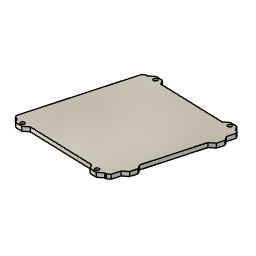
Arc Bed (Mandala) - BETA (Autodesk Fusion 360 design; units mm, degrees)
Autodesk Fusion 360 part; units mm, degrees
note: some values were not read from the file. Set by a fixed rule: which sketch regions a step uses.
sketch "Sketch1" plane through (0, 0, 0) normal (0, 0, 1) x (1, 0, 0) in component "Precision Alca5/ATP5/MIC6/5083 Aluminum Bed Plate"
  line L0 (92.5, -92.5) -> (-92.5, -92.5)
  line L1 (-92.5, -92.5) -> (-92.5, 92.5)
  line L2 (92.5, 92.5) -> (92.5, -92.5)
  line L3 (92.5, -92.5) -> (-92.5, 92.5) construction
  line L4 (-92.5, -92.5) -> (92.5, 92.5) construction
  line L5 (-88.5, 92.5) -> (-92.5, 88.5)
  line L6 (88.5, 92.5) -> (92.5, 88.5)
  line L7 (72.5, -72.5) -> (-72.5, -72.5) construction
  line L8 (-72.5, -72.5) -> (-72.5, 72.5) construction
  line L9 (-72.5, 72.5) -> (72.5, 72.5) construction
  line L10 (72.5, 72.5) -> (72.5, -72.5) construction
  line L11 (72.5, -72.5) -> (-72.5, 72.5) construction
  line L12 (-72.5, -72.5) -> (72.5, 72.5) construction
  circle A0 centre (72.5, 72.5) radius 9.575
  circle A1 centre (-72.5, 72.5) radius 9.575
  circle A2 centre (-72.5, -72.5) radius 9.575
  circle A3 centre (72.5, -72.5) radius 9.575
  line L13 (-92.5, -92.5) -> (-92.5, -99.5)
  line L14 (-92.5, -99.5) -> (92.5, -99.5)
  line L15 (92.5, -99.5) -> (92.5, -92.5)
  line L16 (-92.5, -74.5) -> (-67.5, -99.5)
  line L17 (92.5, -74.5) -> (67.5, -99.5)
  line L18 (-55.5, -99.5) -> (-48.5, -92.5)
  line L19 (55.5, -99.5) -> (48.5, -92.5)
  line L20 (-92.5, -88.5) -> (-88.5, -92.5)
  line L21 (92.5, -88.5) -> (88.5, -92.5)
  line L22 (90, 90) -> (-90, 90)
  line L23 (-90, 90) -> (-90, -90)
  line L24 (-90, -90) -> (90, -90)
  line L25 (90, -90) -> (90, 90)
  line L26 (90, 90) -> (-90, -90) construction
  line L27 (-90, 90) -> (90, -90) construction
  line L28 (-89.5, -89.5) -> (89.5, -89.5)
  line L29 (89.5, -89.5) -> (89.5, 89.5)
  line L30 (89.5, 89.5) -> (-89.5, 89.5)
  line L31 (-89.5, 89.5) -> (-89.5, -89.5)
  line L32 (-70, 90) -> (-70, 89.5)
  line L33 (-89.5, 70) -> (-90, 70)
  line L34 (-90, -70) -> (-89.5, -70)
  line L35 (-70, -89.5) -> (-70, -90)
  line L36 (70, -89.5) -> (70, -90)
  line L37 (89.5, -70) -> (90, -70)
  line L38 (70, 90) -> (70, 89.5)
  line L39 (89.5, 70) -> (90, 70)
  line L40 (-92.5, 72.5) -> (-99.5, 72.5) construction
  line L41 (-99.5, 78.5) -> (-99.5, 66.5)
  line L42 (-99.5, 78.5) -> (-92.5, 85.5)
  line L43 (-92.5, 72.5) -> (-72.5, 72.5) construction
  line L44 (-92.5, 59.5) -> (-99.5, 66.5)
  circle A4 centre (-94.05, 72.5) radius 1.55
  line L45 (-72.5, 0) -> (72.5, 0)
  line L46 (0, 72.5) -> (0, -72.5)
  circle A5 centre (-94.05, 72.5) radius 3.1
  circle A6 centre (-94.05, -72.5) radius 1.55
  circle A7 centre (-94.05, -72.5) radius 3.1
  line L47 (-92.5, -59.5) -> (-99.5, -66.5)
  line L48 (-99.5, -78.5) -> (-99.5, -66.5)
  line L49 (-99.5, -78.5) -> (-92.5, -85.5)
  circle A8 centre (94.05, -72.5) radius 1.55
  circle A9 centre (94.05, -72.5) radius 3.1
  line L50 (99.5, -78.5) -> (99.5, -66.5)
  line L51 (99.5, -78.5) -> (92.5, -85.5)
  line L52 (92.5, -59.5) -> (99.5, -66.5)
  circle A10 centre (94.05, 72.5) radius 1.55
  circle A11 centre (94.05, 72.5) radius 3.1
  line L53 (92.5, 59.5) -> (99.5, 66.5)
  line L54 (99.5, 78.5) -> (99.5, 66.5)
  line L55 (99.5, 78.5) -> (92.5, 85.5)
  circle A12 centre (-72.5, 0) radius 9.575
  circle A13 centre (0, 0) radius 9.575
  circle A14 centre (0, 72.5) radius 9.575
  circle A15 centre (72.5, 0) radius 9.575
  circle A16 centre (0, -72.5) radius 9.575
  line L56 (-1.6, 25.2701) -> (-1.6, 28.4701) construction
  line L57 (-1.6, 28.4701) -> (1.6, 28.4701) construction
  line L58 (1.6, 25.2701) -> (-1.6, 28.4701) construction
  line L59 (-1.6, 25.2701) -> (1.6, 28.4701) construction
  line L60 (92.5, 92.5) -> (-88.5, 92.5)
  line L61 (1.6, 28.4701) -> (1.6, 25.2701) construction
  line L62 (-1.6, 25.2701) -> (1.6, 25.2701) construction
  circle A17 centre (0, 26.8701) radius 2.2627
  line L63 (0, 26.8701) -> (-65.6299, 92.5) construction
  circle A18 centre (-11.3137, 38.1838) radius 2.2627
  line L64 (-1.6, 25.2701) -> (-12.9137, 36.5838)
  line L65 (1.6, 28.4701) -> (-9.7137, 39.7838)
  line L66 (-92.5, 92.5) -> (-88.5, 92.5)
  line L67 (-13.4561, 38.9119) -> (-67.0442, 92.5)
  line L68 (-12.0419, 40.3261) -> (-64.2157, 92.5)
  point P0 (0, 26.8701)
  dimension "d434_1" = 185
  dimension "d435_1" = 185
  dimension "d437_1" = 4
  dimension "d438_1" = 4
  dimension "d443_1" = 145
  dimension "d444_1" = 145
  dimension "d445_1" = 19.15
  dimension "d448_1" = 19.15
  dimension "d451_1" = 19.15
  dimension "d452_1" = 19.15
  dimension "d471_1" = 7
  dimension "d472_1" = 25
  dimension "d473_1" = 25
  dimension "d479_1" = 12
  dimension "d480_1" = 12
  dimension "d481_1" = 135
  dimension "d482_1" = 135
  dimension "d561_1" = 4
  dimension "d562_1" = 4
  dimension "d574_1" = 180
  dimension "d575_1" = 180
  dimension "d577_1" = 20
  dimension "d578_1" = 20
  dimension "d581_1" = 20
  dimension "d582_1" = 20
  dimension "d583_1" = 20
  dimension "d584_1" = 20
  dimension "d585_1" = 20
  dimension "d586_1" = 20
  dimension "d607_1" = 7
  dimension "d608_1" = 12
  dimension "d610_1" = 45
  dimension "d611_1" = 45
  dimension "d612_1" = 3.1
  dimension "d614_1" = 6.2
  dimension "d615_1" = 19.15
  dimension "d616_1" = 19.15
  dimension "d617_1" = 19.15
  dimension "d618_1" = 19.15
  dimension "d619_1" = 19.15
  dimension "d74" = 3.2
  dimension "d75" = 3.2
  dimension "d90" = 16
  dimension "d98" = 185
  dimension "d99" = 185
  dimension "d103" = 1
  dimension "d104" = 1
  dimension "d105" = 18
  dimension "d108" = 45
  constraint horizontal L0
  constraint perpendicular L0 L1
  constraint parallel L1 L2
  constraint coincident L3 A13.centre
  constraint coincident L4 A13.centre
  constraint coincident A13.centre origin
  constraint coincident L1 L5.end
  constraint perpendicular L3 L5
  constraint coincident L2 L6.end
  constraint perpendicular L4 L6
  constraint horizontal L7
  constraint perpendicular L7 L8
  constraint parallel L7 L9
  constraint parallel L8 L10
  constraint coincident L11 A13.centre
  constraint coincident L12 A13.centre
  constraint coincident L9.end L10.start
  constraint coincident L8.end L9.start
  constraint coincident L7.end L8.start
  constraint coincident L7.start L10.end
  constraint perpendicular L0 L13
  constraint perpendicular L13 L14
  constraint perpendicular L0 L15
  constraint coincident L0.start L2.end
  constraint coincident L1 L16.start
  constraint coincident L14 L16.end
  constraint perpendicular L4 L16
  constraint coincident L2 L17.start
  constraint coincident L14 L17.end
  constraint perpendicular L3 L17
  constraint coincident L14 L18.start
  constraint coincident L14 L19.start
  constraint coincident L0 L19.end
  constraint coincident L0 L18.end
  constraint coincident L1 L20.start
  constraint coincident L0 L20.end
  constraint perpendicular L4 L20
  constraint coincident L2 L21.start
  constraint coincident L0 L21.end
  constraint perpendicular L3 L21
  constraint horizontal L22
  constraint perpendicular L22 L23
  constraint parallel L22 L24
  constraint parallel L23 L25
  constraint coincident L26 A13.centre
  constraint coincident L27 A13.centre
  constraint coincident L22 L32.start
  constraint coincident L30 L32.end
  constraint perpendicular L30 L32
  constraint coincident L31 L33.start
  constraint coincident L23 L33.end
  constraint perpendicular L23 L33
  constraint coincident L23 L34.start
  constraint coincident L31 L34.end
  constraint perpendicular L31 L34
  constraint coincident L28 L35.start
  constraint coincident L24 L35.end
  constraint perpendicular L24 L35
  constraint coincident L28 L36.start
  constraint coincident L24 L36.end
  constraint perpendicular L24 L36
  constraint coincident L29 L37.start
  constraint coincident L25 L37.end
  constraint perpendicular L25 L37
  constraint coincident L22 L38.start
  constraint coincident L30 L38.end
  constraint perpendicular L30 L38
  constraint coincident L29 L39.start
  constraint coincident L25 L39.end
  constraint perpendicular L25 L39
  constraint coincident L1 L40.start
  constraint perpendicular L1 L40
  constraint vertical L41
  constraint midpoint L40.end L41
  constraint coincident L1 L42.end
  constraint perpendicular L1 L43
  constraint coincident L1 L44.start
  constraint coincident L40 A4.centre
  constraint midpoint L8 L45.start
  constraint midpoint L10 L45.end
  constraint midpoint L9 L46.start
  constraint midpoint L7 L46.end
  constraint concentric A4 A5
  constraint symmetric L41.start L45 L48.start
  constraint symmetric L41.end L45 L47.end
  constraint symmetric L42.end L45 L49.end
  constraint symmetric L44.start L45 L47.start
  constraint symmetric A4 L45 A6
  constraint symmetric L45 A5 A7
  constraint symmetric L41.start L46 L54.start
  constraint symmetric L41.end L46 L53.end
  constraint symmetric L42.end L46 L55.end
  constraint symmetric L44.start L46 L53.start
  constraint symmetric A4 L46 A10
  constraint symmetric L46 A5 A11
  constraint symmetric L46 A6 A8
  constraint symmetric L46 A7 A9
  constraint symmetric L46 L47.start L52.start
  constraint symmetric L46 L47.end L50.end
  constraint symmetric L46 L48.start L50.start
  constraint symmetric L46 L49.end L51.end
  constraint coincident L45.start A12.centre
  constraint coincident L46.start A14.centre
  constraint coincident L45.end A15.centre
  constraint coincident L46.end A16.centre
  constraint tangent L1 A4
  constraint coincident L58 P0
  constraint coincident L59 P0
  constraint coincident L46 P0
  constraint perpendicular L2 L60
  constraint perpendicular L57 L61
  constraint coincident L58.start L61.end
  constraint perpendicular L56 L62
  constraint vertical L61
  constraint vertical L56
  constraint coincident P0 A17.centre
  constraint coincident L57.end A17
  constraint coincident L63 A18.centre
  constraint coincident A17 L56.start
  constraint tangent A17 L64
  constraint coincident A18 L64.end
  constraint tangent A18 L64
  constraint coincident A17 L57.end
  constraint tangent A17 L65
  constraint coincident A18 L65.end
  constraint tangent A18 L65
  constraint parallel L64 L65
  constraint perpendicular L1 L66
  constraint coincident L5.start L60.end
  constraint coincident L60 L63.end
  constraint coincident A18 L67.start
  constraint parallel L63 L67
  constraint coincident A18 L68.start
  constraint parallel L63 L68
  constraint coincident L60 L68.end
  constraint coincident L60 L67.end
  measures "d434_1" distance of L1.end L2.start
  measures "d435_1" distance of L0.end L1.end
  measures "d437_1" distance of L1.end L5.start
  measures "d438_1" distance of L2.start L6.start
  measures "d443_1" distance of L8.end L9.end
  measures "d444_1" distance of L7.end L8.end
  measures "d445_1" diameter of A0
  measures "d448_1" diameter of A1
  measures "d451_1" diameter of A2
  measures "d452_1" diameter of A3
  measures "d471_1" distance of L0.end L13.end
  measures "d472_1" horizontal distance of L17.start L17.end
  measures "d473_1" distance of L1 L16.end
  measures "d479_1" distance of L17.end L19.start
  measures "d480_1" distance of L16.end L18.start
  measures "d481_1" angle of L14 L18
  measures "d482_1" angle of L14 L19
  measures "d561_1" distance of L0.start L21.end
  measures "d562_1" distance of L0.end L20.end
  measures "d574_1" distance of L23.end L24.end
  measures "d575_1" distance of L22.end L23.end
  measures "d577_1" distance of L22.end L32
  measures "d578_1" distance of L22.end L33
  measures "d581_1" distance of L23.end L34
  measures "d582_1" distance of L23.end L35
  measures "d583_1" distance of L24.end L36
  measures "d584_1" distance of L24.end L37
  measures "d585_1" distance of L22.start L38
  measures "d586_1" distance of L22.start L39
  measures "d607_1" distance of L40.start L40.end
  measures "d608_1" distance of L41.start L41.end
  measures "d610_1" angle of L1 L42
  measures "d611_1" angle of L1 L44
  measures "d612_1" diameter of A4
  measures "d614_1" diameter of A5
  measures "d615_1" diameter of A12
  measures "d616_1" diameter of A13
  measures "d617_1" diameter of A14
  measures "d618_1" diameter of A15
  measures "d619_1" diameter of A16
  measures "d74" distance of L56.end L57.end
  measures "d75" distance of L56.start L56.end
  measures "d90" distance of P0 A18.centre
  measures "d98" distance of L0 L60
  measures "d99" distance of L1 L2
  measures "d103" distance of L63 L68
  measures "d104" distance of L63 L67
  measures "d105" distance of L8.end L67
  measures "d108" angle of L60 L68
extrude "Extrude1" add sketch "Sketch1" against normal blind 6.35 contours L0 L2 L17 L21 L24 L25 A9 | L0 L14 L17 L19 | L0 L16 L17 L24 | L2 A9 L50 L51 L52 | L17 L24 L28 L36 | L17 L24 L25 L28 L29 | L2 L17 A9 | L2 A9 | L0 L14 L16 L18 | L16 L17 L28 L29 L30 L31 A17 A18 L64 L65 L67 L68 | L17 L28 L29 | L24 L28 L35 L36 | L2 L17 A9 | L2 L6 L17 L22 L25 A9 A11 L60 L68 | L0 L1 L16 L20 L23 L24 A7 | L17 L25 L29 L37 | L16 L24 L28 L35 | L16 L23 L24 L28 L31 | L25 L29 L37 L39 | L2 A11 L53 L54 L55 | L16 L28 L31 | L22 L25 L29 L30 L38 L39 | L2 A11 | L2 A11 | L1 A7 L47 L48 L49 | L16 L23 L31 L34 | L1 L5 L16 L22 L23 A5 A7 L60 L67 | L1 A7 | L1 L16 A7 | L23 L31 L33 L34 | L1 L16 A7 | L22 L30 L38 L68 | L22 L23 L30 L31 L32 L33 | L30 A18 L67 L68 | L22 L30 L67 L68 | L22 L60 L67 L68 | L22 L30 L32 L67 | A18 | L1 L41 L42 L44 A5 | L46 A17 A18 L64 L65 | L1 A5 | L1 A5 | L46 A17 L65 | L46 A17 | L46 A17 | A0 | A1 | A2 | A3 | L45 L46 A13 | L45 L46 A13 | L45 L46 A13 | L45 L46 A13 | A12 | A14 | A15 | A16 in component "Precision Alca5/ATP5/MIC6/5083 Aluminum Bed Plate"
extrude "Extrude6" cut sketch "Sketch1" along normal blind 3.2 from surface at -6.35 contours A18 | L46 A17 A18 L64 L65 | L46 A17 L65 | L46 A17 | L46 A17 in component "Precision Alca5/ATP5/MIC6/5083 Aluminum Bed Plate"
extrude "Extrude7" cut sketch "Sketch1" along normal blind 2 from surface at -6.35 contours L30 A18 L67 L68 | L22 L30 L67 L68 | L22 L60 L67 L68 in component "Precision Alca5/ATP5/MIC6/5083 Aluminum Bed Plate"
fillet "Fillet2" radius 0.6 2 edges at (-67.0442, 92.5, -5.35) (-64.2157, 92.5, -5.35) in component "Precision Alca5/ATP5/MIC6/5083 Aluminum Bed Plate"
hole "Hole2" at (-94.05, -72.5, 0) at (-94.05, 72.5, 0) at (94.05, 72.5, 0) at (94.05, -72.5, 0) direction (0, 0, -1) diameter 3.2 depth 6.35 tip angle 180 counterbore diameter 6.5 counterbore depth 3 in component "Precision Alca5/ATP5/MIC6/5083 Aluminum Bed Plate"
extrude "Extrude2" cut sketch "Sketch1" along normal blind 0.2 from surface at -6.35 contours L17 L24 L28 L36 | L17 L24 L25 L28 L29 | L17 L25 L29 L37 | L16 L24 L28 L35 | L16 L23 L24 L28 L31 | L22 L25 L29 L30 L38 L39 | L16 L23 L31 L34 | L22 L23 L30 L31 L32 L33 in component "Precision Alca5/ATP5/MIC6/5083 Aluminum Bed Plate"
fillet "Fillet1" radius 0.25 20 edges at (89.5, -89.5, -6.25) (89.5, -70, -6.25) (90, -70, -6.25) (70, -89.5, -6.25) (70, -90, -6.25) (-70, -90, -6.25) (-70, -89.5, -6.25) (-89.5, -89.5, -6.25) (-89.5, -70, -6.25) (-90, -70, -6.25) (-70, 90, -6.25) (-70, 89.5, -6.25) (-89.5, 89.5, -6.25) (-89.5, 70, -6.25) (-90, 70, -6.25) (70, 89.5, -6.25) (70, 90, -6.25) (89.5, 89.5, -6.25) (90, 70, -6.25) (89.5, 70, -6.25) in component "Precision Alca5/ATP5/MIC6/5083 Aluminum Bed Plate"
fillet "Fillet1" radius 0.5 4 edges at (90, -90, -6.25) (90, 90, -6.25) (-90, 90, -6.25) (-90, -90, -6.25) in component "Precision Alca5/ATP5/MIC6/5083 Aluminum Bed Plate"
component "Assembly" placed x (1, 0, 0) y (0, 1, 0) z (0, 0, 1) at (0, 0, 0)
component "Precision Alca5/ATP5/MIC6/5083 Aluminum Bed Plate" placed x (1, 0, 0) y (0, 1, 0) z (0, 0, 1) at (0, 0, 0) in component "Assembly"
equation "d434_1 = bed_border_width + bed_width"
equation "d435_1 = bed_border_width + bed_depth"
equation "d437_1 = bed_milling_chamfer_size"
equation "d438_1 = bed_milling_chamfer_size"
equation "d443_1 = bed_mounting_hole_spacing_x"
equation "d444_1 = bed_mounting_hole_spacing_y"
equation "d445_1 = magnet_inset_diameter"
equation "d448_1 = magnet_inset_diameter"
equation "d451_1 = magnet_inset_diameter"
equation "d452_1 = magnet_inset_diameter"
equation "d455_1 = -bed_thickness"
equation "d471_1 = bed_ridge_size"
equation "d472_1 = bed_ridge_angle_width"
equation "d473_1 = bed_ridge_angle_width"
equation "d479_1 = bed_ridge_grip_width"
equation "d480_1 = bed_ridge_grip_width"
equation "d481_1 = 45 deg + 45 deg + 45 deg"
equation "d482_1 = 45 deg + 45 deg + 45 deg"
equation "d561_1 = bed_milling_chamfer_size"
equation "d562_1 = bed_milling_chamfer_size"
equation "d574_1 = silicone_heater_width"
equation "d575_1 = silicone_heater_depth"
equation "d576_1 = -silicone_heater_marking_width"
equation "d577_1 = silicone_heater_marking_size"
equation "d578_1 = silicone_heater_marking_size"
equation "d581_1 = silicone_heater_marking_size"
equation "d582_1 = silicone_heater_marking_size"
equation "d583_1 = silicone_heater_marking_size"
equation "d584_1 = silicone_heater_marking_size"
equation "d585_1 = silicone_heater_marking_size"
equation "d586_1 = silicone_heater_marking_size"
equation "d587_1 = -bed_thickness"
equation "d591_1 = silicone_heater_marking_width / 2"
equation "d593_1 = silicone_heater_marking_width"
equation "d607_1 = bed_ridge_size"
equation "d608_1 = bed_ridge_grip_width"
equation "d615_1 = magnet_inset_diameter"
equation "d616_1 = magnet_inset_diameter"
equation "d617_1 = magnet_inset_diameter"
equation "d618_1 = magnet_inset_diameter"
equation "d619_1 = magnet_inset_diameter"
equation "d620_1 = bed_thickness"
equation "metal_chamfer_size = 0.6 mm" comment "The size of the chamfer when applied to metal parts, for deburring"
equation "bed_width = 180 mm"
equation "bed_depth = 180 mm"
equation "bed_thickness = 6.35 mm"
equation "bed_border_width = 5 mm"
equation "bed_milling_chamfer_size = 4 mm"
equation "bed_mounting_hole_spacing_y = bed_depth - bed_mounting_hole_spacing_inset"
equation "bed_mounting_hole_spacing_x = bed_width - bed_mounting_hole_spacing_inset"
equation "bed_screw_hole_diameter = 3.1 mm"
equation "bed_mounting_hole_spacing_inset = 35 mm"
equation "bed_ridge_size = 7 mm"
equation "bed_ridge_angle_width = 25 mm"
equation "bed_ridge_grip_width = 12 mm"
equation "silicone_heater_marking_size = 20 mm"
equation "silicone_heater_marking_width = 0.5 mm"
equation "silicone_heater_thickness = 2 mm"
equation "silicone_heater_fillet_radius = 1 mm"
equation "magnet_inset_diameter = 19.15 mm"
equation "magnet_inset_depth = 3.175 mm + 0.1 mm"
equation "magnet_chamfer_size = 0.3 mm"
equation "silicone_heater_width = 180 mm"
equation "silicone_heater_depth = 180 mm"
equation "d74 = thermistor_inset_thickness"
equation "d75 = thermistor_inset_thickness"
equation "thermistor_inset_thickness = 3.2 mm"
equation "d81 = -bed_thickness"
equation "d82 = thermistor_inset_thickness"
equation "thermistor_inset_wire_thickness = 2 mm"
equation "d98 = bed_border_width + bed_depth"
equation "d99 = bed_border_width + bed_width"
equation "d100 = -bed_thickness"
equation "d101 = thermistor_inset_wire_thickness"
equation "d103 = thermistor_inset_wire_thickness / 2"
equation "d104 = thermistor_inset_wire_thickness / 2"
equation "d107 = metal_chamfer_size"
